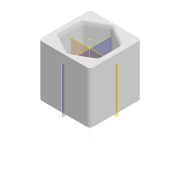
# Autodesk Inventor part: 30_Laser_to_M12Adapter
Saved by Autodesk Inventor 2022 (Build 260153000, 153)
## iProperties
Created: 2023-02-07
Part Number: 30_Laser_to_M12Adapter
Material: Generisch
Document SubType Name: Modeling
Designer: diederichbenedict
Density: 1 g/cm^3
Appearance: Vorgabe
Author: diederichbenedict
Autodesk Inventor part; units mm, degrees
ref_plane "YZ Plane" through (0, 0, 0) normal (1, 0, 0) x (0, 1, 0)
ref_plane "XZ Plane" through (0, 0, 0) normal (0, 1, 0) x (-1, 0, 0)
ref_plane "XY Plane" through (0, 0, 0) normal (0, 0, 1) x (1, 0, 0)
sketch "Skizze1" plane through (0, 0, 0) normal (0, 1, 0) x (-1, 0, 0)
  line L0 (6.725, 3.8827) -> (6.725, -3.8827)
  line L1 (6.725, -3.8827) -> (0, -7.7654)
  line L2 (0, -7.7654) -> (-6.725, -3.8827)
  line L3 (-6.725, -3.8827) -> (-6.725, 3.8827)
  line L4 (-6.725, 3.8827) -> (0, 7.7654)
  line L5 (0, 7.7654) -> (6.725, 3.8827)
  line L6 (-8, -8) -> (8, -8)
  line L7 (8, -8) -> (8, 8)
  line L8 (8, 8) -> (-8, 8)
  line L9 (-8, 8) -> (-8, -8)
  line L10 (-8, -8) -> (8, 8) construction
  line L11 (8, -8) -> (-8, 8) construction
  point P0 (0, 0)
  point P1 (0, 0)
  point P2 (-0.3096, 7.5)
  point P3 (-0.3096, -7.5)
  point P4 (0.3096, -7.5)
  point P5 (0.3096, 7.5)
  dimension "d0" = 16
  dimension "d1" = 16
  dimension "d2" = 13.45
  constraints: 24 end point, 3 parallel, 2 midpoint, 1 coincident, 1 horizontal, 1 perpendicular, 13 other
  measures "d0" distance of L8.end L7.end
  measures "d1" distance of L7.end L6.end
  measures "d2" distance between parallel lines of L3 L0
extrude "Extrusion1" add sketch "Skizze1" along normal blind 3
fillet "Rundung1" radius 2 6 edges at (-6.725, 1.5, -3.8827) (-6.725, 1.5, 3.8827) (0, 1.5, 7.7654) (6.725, 1.5, 3.8827) (6.725, 1.5, -3.8827) (0, 1.5, -7.7654)
sketch "Skizze2" plane through (0, 3, 0) normal (0, 1, 0) x (1, 0, 0)
  line L0 (-8, 8) -> (-8, -8) projected
  line L1 (-8, -8) -> (8, -8) projected
  line L2 (8, -8) -> (8, 8) projected
  line L3 (8, 8) -> (-8, 8) projected
  line L4 (-5.725, 4.46) -> (-1, 7.188) projected
  arc A0 (1, 7.188) -> (-1, 7.188) centre (0, 5.456) ccw projected
  line L5 (1, 7.188) -> (5.725, 4.46) projected
  arc A1 (6.725, 2.728) -> (5.725, 4.46) centre (4.725, 2.728) ccw projected
  line L6 (6.725, 2.728) -> (6.725, -2.728) projected
  arc A2 (5.725, -4.46) -> (6.725, -2.728) centre (4.725, -2.728) ccw projected
  line L7 (5.725, -4.46) -> (1, -7.188) projected
  arc A3 (-1, -7.188) -> (1, -7.188) centre (0, -5.456) ccw projected
  line L8 (-1, -7.188) -> (-5.725, -4.46) projected
  arc A4 (-6.725, -2.728) -> (-5.725, -4.46) centre (-4.725, -2.728) ccw projected
  line L9 (-6.725, -2.728) -> (-6.725, 2.728) projected
  arc A5 (-5.725, 4.46) -> (-6.725, 2.728) centre (-4.725, 2.728) ccw projected
  line L10 (0, -6.8416) -> (-5.925, -3.4208)
  line L11 (-5.925, -3.4208) -> (-5.925, 3.4208)
  line L12 (-5.925, 3.4208) -> (0, 6.8416)
  line L13 (0, 6.8416) -> (5.925, 3.4208)
  line L14 (5.925, 3.4208) -> (5.925, -3.4208)
  line L15 (5.925, -3.4208) -> (0, -6.8416)
  point P0 (0, 0)
  point P1 (0, 0)
  point P2 (8, 5.7735)
  point P3 (8, -5.7735)
  point P4 (-8, -5.7735)
  point P5 (-8, 5.7735)
  point P6 (4.1436, -8)
  point P7 (-4.1436, -8)
  point P8 (4.1436, 8)
  point P9 (-4.1436, 8)
  dimension "d6" = 11.85
  constraints: 12 end point, 1 coincident, 13 other
  measures "d6" distance between parallel lines of L14 L11
extrude "Extrusion2" add sketch "Skizze2" along normal blind 13 contours L3 L2 L1 L0 | L4 A0 L5 A1 L6 A2 L7 A3 L8 A4 L9 A5
fillet "Rundung2" radius 1 16 edges at (0, 9.5, 6.8416) (-5.925, 9.5, 3.4208) (-5.925, 9.5, -3.4208) (0, 9.5, -6.8416) (5.925, 9.5, -3.4208) (5.925, 9.5, 3.4208) (8, 8, -8) (-8, 8, -8) (-8, 8, 8) (8, 8, 8) (-2.9625, 16, -5.1312) (-5.925, 16, 0) (-2.9625, 16, 5.1312) (2.9625, 16, 5.1312) (5.925, 16, 0) (2.9625, 16, -5.1312)
ref_plane "Arbeitsebene1" through (0, 0, -8) normal (-1, 0, 0) x (0, 0, 1)
ref_plane "Arbeitsebene2" through (-8, 0, 0) normal (0, 0, 1) x (1, 0, 0)
sketch "Skizze3" plane through (0, 16, 0) normal (0, 1, 0) x (1, 0, 0)
  arc A0 (7, -8) -> (8, -7) centre (7, -7) ccw projected
  line L0 (8, -7) -> (8, 7) projected
  arc A1 (8, 7) -> (7, 8) centre (7, 7) ccw projected
  line L1 (7, 8) -> (-7, 8) projected
  arc A2 (-7, 8) -> (-8, 7) centre (-7, 7) ccw projected
  line L2 (-8, 7) -> (-8, -7) projected
  arc A3 (-8, -7) -> (-7, -8) centre (-7, -7) ccw projected
  line L3 (-7, -8) -> (7, -8) projected
  arc A4 (-1, -7.419) -> (1, -7.419) centre (0, -5.6869) ccw projected
  line L4 (-5.925, -4.5755) -> (-1, -7.419) projected
  arc A5 (-6.925, -2.8435) -> (-5.925, -4.5755) centre (-4.925, -2.8435) ccw projected
  line L5 (-6.925, 2.8435) -> (-6.925, -2.8435) projected
  arc A6 (-5.925, 4.5755) -> (-6.925, 2.8435) centre (-4.925, 2.8435) ccw projected
  line L6 (-1, 7.419) -> (-5.925, 4.5755) projected
  arc A7 (1, 7.419) -> (-1, 7.419) centre (0, 5.6869) ccw projected
  line L7 (5.925, 4.5755) -> (1, 7.419) projected
  arc A8 (6.925, 2.8435) -> (5.925, 4.5755) centre (4.925, 2.8435) ccw projected
  line L8 (6.925, -2.8435) -> (6.925, 2.8435) projected
  arc A9 (5.925, -4.5755) -> (6.925, -2.8435) centre (4.925, -2.8435) ccw projected
  line L9 (1, -7.419) -> (5.925, -4.5755) projected
  line L10 (-8, -5.6869) -> (8, -5.6869)
  line L11 (8, -5.6869) -> (8, -13.6869)
  line L12 (6, -15.6869) -> (-6, -15.6869)
  line L13 (-8, -13.6869) -> (-8, -5.6869)
  circle A10 centre (-4.925, -12.0977) radius 1.4
  circle A11 centre (4.925, -12.0977) radius 1.4
  arc A12 (-8, -13.6869) -> (-6, -15.6869) centre (-6, -13.6869) ccw
  arc A13 (6, -15.6869) -> (8, -13.6869) centre (6, -13.6869) ccw
  point P0 (0, 0)
  point P1 (8, -15.6869)
  point P2 (8, -7)
  dimension "d10" = 10
  dimension "d11" = 2.8
  dimension "d12" = 2.8
  dimension "d13" = 2
  constraints: 8 end point, 4 centre point, 4 point on circle, 4 tangent, 3 point on line, 2 parallel, 1 equal radius, 1 horizontal, 1 perpendicular
  measures "d10" distance of L10.end point (8, -15.687)
  measures "d11" diameter of A10
  measures "d12" diameter of A11
  measures "d13" radius of A12
extrude "Extrusion3" add sketch "Skizze3" against normal blind 3 contours A0 L11 A13 L12 A12 L13 A3 L3
